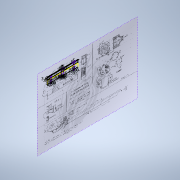
# Autodesk Inventor part: Part1
Saved by Autodesk Inventor 2021 (Build 250183000, 183)
## iProperties
Created: 2021-08-19
Part Number: Part1
Material: Generic
Document SubType Name: Modeling
Designer: newic
Density: 1 g/cm^3
Appearance: Default
Author: newic
Autodesk Inventor part; units mm, degrees
ref_plane "YZ Plane" through (0, 0, 0) normal (1, 0, 0) x (0, 1, 0)
ref_plane "XZ Plane" through (0, 0, 0) normal (0, 1, 0) x (-1, 0, 0)
ref_plane "XY Plane" through (0, 0, 0) normal (0, 0, 1) x (1, 0, 0)
sketch "Sketch1" plane through (0, 0, 0) normal (0, 1, 0) x (-1, 0, 0)
  line L0 (0, 0) -> (139.7, 0)
  line L1 (139.7, 0) -> (139.7, -920.75)
  line L2 (139.7, -920.75) -> (0, -920.75)
  line L3 (0, -920.75) -> (0, 0)
  dimension "d0" = 139.7
  dimension "d1" = 920.75
  constraints: 8 end point, 2 parallel, 1 horizontal, 1 perpendicular
  measures "d0" distance of L1.end L2.end
  measures "d1" distance of L0.end L1.end
extrude "Extrusion1" add sketch "Sketch1" along normal blind 100.33
sketch "Sketch2" plane through (0, 0, 0) normal (1, 0, 0) x (0, 0, -1)
  line L0 (920.75, 0) -> (0, 0) projected
  line L1 (0, 0) -> (920.75, 0)
  line L2 (-297.6389, 409.8513) -> (2710.7909, 409.8513) construction
  line L3 (2710.7909, 409.8513) -> (2710.7909, -1716.9746) construction
  line L4 (2710.7909, -1716.9746) -> (-297.6389, -1716.9746) construction
  line L5 (-297.6389, -1716.9746) -> (-297.6389, 409.8513) construction
  line L6 (0, 0) -> (920.75, 0) projected
  line L7 (920.75, 0) -> (920.75, 100.33) projected
  line L8 (0, 100.33) -> (920.75, 100.33) projected
  line L9 (0, 0) -> (0, 100.33) projected
  line L10 (0, 100.33) -> (0, 120.65)
  line L11 (0, 120.65) -> (920.75, 120.65)
  line L12 (920.75, 120.65) -> (920.75, 100.33)
  line L13 (0, 120.65) -> (0, 196.85)
  line L14 (0, 196.85) -> (920.75, 196.85)
  line L15 (920.75, 196.85) -> (920.75, 120.65)
  line L16 (477.9962, 0) -> (477.9962, -13.97)
  line L17 (477.9962, -13.97) -> (434.8162, -13.97)
  line L18 (434.8162, -13.97) -> (434.8162, 0)
  line L19 (133.294, 0) -> (133.294, -13.97)
  line L20 (133.294, -13.97) -> (90.114, -13.97)
  line L21 (90.114, -13.97) -> (90.114, 0)
  line L22 (769.0257, 0) -> (769.0257, -13.97)
  line L23 (769.0257, -13.97) -> (812.2057, -13.97)
  line L24 (812.2057, -13.97) -> (812.2057, 0)
  line L25 (456.4062, 196.85) -> (456.4062, 176.53)
  line L26 (456.4062, 176.53) -> (957.4766, 176.53)
  line L27 (456.4062, 176.53) -> (-70.4596, 176.53)
  line L28 (434.8162, 176.53) -> (434.8162, 184.15)
  line L29 (477.9962, 176.53) -> (477.9962, 184.15)
  line L30 (434.8162, -13.97) -> (477.9962, -13.97)
  line L31 (477.9962, -13.97) -> (477.9962, 184.15)
  line L32 (434.8162, 184.15) -> (434.8162, -13.97)
  line L33 (769.0257, -13.97) -> (812.2057, -13.97)
  line L34 (812.2057, -13.97) -> (812.2057, 184.15)
  line L35 (769.0257, 184.15) -> (769.0257, -13.97)
  line L36 (90.114, -13.97) -> (133.294, -13.97)
  line L37 (133.294, -13.97) -> (133.294, 163.83)
  line L38 (133.294, 163.83) -> (90.114, 163.83)
  line L39 (90.114, 163.83) -> (90.114, -13.97)
  line L40 (90.114, -13.97) -> (111.704, -13.97)
  line L41 (111.704, -13.97) -> (100.909, -13.97)
  line L42 (100.909, -13.97) -> (122.499, -13.97)
  line L43 (122.499, -13.97) -> (122.499, -33.02)
  line L44 (122.499, -33.02) -> (100.909, -33.02)
  line L45 (100.909, -33.02) -> (100.909, -13.97)
  line L46 (434.8162, -13.97) -> (456.4062, -13.97)
  line L47 (456.4062, -13.97) -> (445.6112, -13.97)
  line L48 (445.6112, -13.97) -> (467.2012, -13.97)
  line L49 (467.2012, -13.97) -> (467.2012, -33.02)
  line L50 (467.2012, -33.02) -> (445.6112, -33.02)
  line L51 (445.6112, -33.02) -> (445.6112, -13.97)
  line L52 (769.0257, -13.97) -> (790.6157, -13.97)
  line L53 (790.6157, -13.97) -> (779.8207, -13.97)
  line L54 (779.8207, -13.97) -> (801.4107, -13.97)
  line L55 (801.4107, -13.97) -> (801.4107, -33.02)
  line L56 (801.4107, -33.02) -> (779.8207, -33.02)
  line L57 (779.8207, -33.02) -> (779.8207, -13.97)
  line L58 (434.8162, 196.85) -> (434.8162, 203.2)
  line L59 (434.8162, 203.2) -> (495.6691, 203.2)
  line L60 (418.8725, 203.2) -> (503.7191, 203.2)
  line L61 (418.8725, 182.88) -> (503.7191, 182.88)
  line L62 (851.0188, 203.2) -> (730.7071, 203.2)
  line L63 (851.0188, 182.88) -> (730.7071, 182.88)
  line L64 (477.9962, 165.6349) -> (477.9962, 191.9525)
  line L65 (427.1534, 182.88) -> (514.6465, 182.88)
  line L66 (434.8162, 184.15) -> (434.8162, 162.3234)
  line L67 (434.8162, 0) -> (413.2262, 0)
  line L68 (413.2262, 0) -> (413.2262, -11.43)
  line L69 (413.2262, -11.43) -> (371.9512, -11.43)
  line L70 (371.9512, -11.43) -> (371.9512, 67.31)
  dimension "d4" = 920.75
  dimension "d32" = 20.32
  dimension "d33" = 76.2
  dimension "d34" = 13.97
  dimension "d35" = 43.18
  dimension "d36" = 13.97
  dimension "d37" = 43.18
  dimension "d38" = 13.97
  dimension "d39" = 13.97
  dimension "d40" = 43.18
  dimension "d41" = 20.32
  dimension "d42" = 7.62
  dimension "d43" = 7.62
  dimension "d45" = 21.59
  dimension "d46" = 19.05
  dimension "d47" = 21.59
  dimension "d48" = 19.05
  dimension "d49" = 21.59
  dimension "d50" = 19.05
  dimension "d51" = 6.35
  dimension "d52" = 20.32
  dimension "d56" = 20.32
  dimension "d58" = 21.59
  dimension "d59" = 11.43
  dimension "d60" = 41.275
  dimension "d61" = 78.74
  constraints: 124 end point, 20 perpendicular, 14 point on line, 13 parallel, 9 horizontal, 6 midpoint, 3 vertical, 10 other
  measures "d4" distance of L0.start L0.end
  measures "d32" distance of L8.start L10.end
  measures "d33" distance of L10.end L13.end
  measures "d34" distance of L16.start L16.end
  measures "d35" distance of L16.end L17.end
  measures "d36" distance of L19.start L19.end
  measures "d37" distance of L19.end L20.end
  measures "d38" distance of L20.end L21.end
  measures "d39" distance of L22.start L22.end
  measures "d40" distance of L22.end L23.end
  measures "d41" distance of L25.start L25.end
  measures "d42" distance of L28.start L28.end
  measures "d43" distance of L29.start L29.end
  measures "d45" distance of L43.end L44.end
  measures "d46" distance of L42.end L43.end
  measures "d47" distance of L49.end L50.end
  measures "d48" distance of L48.end L49.end
  measures "d49" distance of L55.end L56.end
  measures "d50" distance of L54.end L55.end
  measures "d51" distance of L58.start L58.end
  measures "d52" distance between parallel lines of L60 L61
  measures "d56" distance between parallel lines of L62 L63
  measures "d58" distance of L18.end L67.end
  measures "d59" distance of L67.end L68.end
  measures "d60" distance of L68.end L69.end
  measures "d61" distance of L69.end L70.end
body "Solid1"
